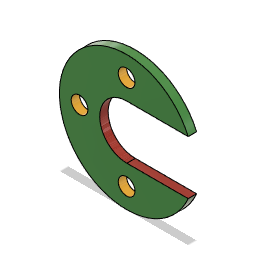
Questão1 (Autodesk Fusion 360 design; units mm, degrees)
Autodesk Fusion 360 part; units mm, degrees
sketch "Sketch1" plane through (0, 0, 0) normal (0, 0, 1) x (1, 0, 0)
  circle A0 centre (-50, 73) radius 5
  circle A1 centre (-50, 17) radius 5
  circle A2 centre (-78, 45) radius 5
  line L0 (-50.0531, 60.9999) -> (-49.9469, 60.9999)
  line L1 (-50.1491, 29.0007) -> (-49.8509, 29.0007)
  arc A3 (-49.9469, 60.9999) -> (-49.8509, 29.0007) centre (-50, 45) ccw
  line L2 (-50.0531, 60.9999) -> (-13.3394, 60.9999)
  line L3 (-13.3391, 29.0007) -> (-50.1491, 29.0007)
  arc A4 (-13.3394, 60.9999) -> (-13.3391, 29.0007) centre (-50, 45) ccw
  dimension "d1" = 80
  dimension "d3" = 10
  dimension "d5" = 10
  dimension "d7" = 10
  constraint concentric A3 A4
  constraint horizontal L0
  constraint coincident L0.start A3
  constraint coincident L1.start A3
  constraint horizontal L1
  constraint horizontal L2
  constraint parallel L1 L3
  measures "d1" diameter of A4
  measures "d3" diameter of A0
  measures "d5" diameter of A1
  measures "d7" diameter of A2
extrude "Extrude1" add sketch "Sketch1" along normal blind 5
